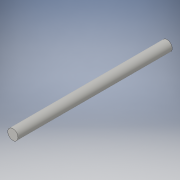
# Autodesk Inventor part: 4x40 Tap
Saved by Autodesk Inventor 2016 (Build 200138000, 138)
## iProperties
Created: 2015-09-21
Part Number: 4x40 Tap
Material: Generic
Document SubType Name: Modeling
Designer: steele
Density: 1 g/cm^3
Appearance: Default
Author: steele
Autodesk Inventor part; units mm, degrees
ref_plane "YZ Plane" through (0, 0, 0) normal (1, 0, 0) x (0, 1, 0)
ref_plane "XZ Plane" through (0, 0, 0) normal (0, 1, 0) x (-1, 0, 0)
ref_plane "XY Plane" through (0, 0, 0) normal (0, 0, 1) x (1, 0, 0)
sketch "Sketch1" plane through (0, 0, 0) normal (0, 0, 1) x (1, 0, 0)
  circle A0 centre (0, 0) radius 2.54
  dimension "d2" = 5.08
  constraints: 1 centre point, 1 coincident
  measures "d2" diameter of A0
extrude "Extrusion1" add sketch "Sketch1" along normal mid plane 76.2
equation "\"d2\" = tapDiam4x40"
equation "\"d0\" = tapLength4x40"
equation "\"tapDiam1d4x28\" = 5.08"
equation "\"tapDiam1d4x20\" = 5.08"
equation "\"tapDiam12x24\" = 5.08"
equation "\"tapDiam8x36\" = 5.08"
equation "\"tapDiam10x32\" = 5.08"
equation "\"tapLength4x40\" = 76.2"
equation "\"tapDiam8x32\" = 5.08"
equation "\"lowerCaseHeight\" = 127"
equation "\"tapDiam4x40\" = 5.08"
equation "\"fingerWidth\" = 19.05"
equation "\"lowerCaseDepth\" = 25.4"
equation "\"tapLength6x32\" = 76.2"
equation "\"lowerCaseWidth\" = 254"
equation "\"tapDiam12x28\" = 5.08"
equation "\"tapDiam6x32\" = 5.08"
equation "\"tapDiam6x40\" = 5.08"
equation "\"tapDiam10x24\" = 5.08"
equation "\"tapDiaam4x48\" = 5.08"
equation "\"tapLength4x48\" = 76.2"
body "Solid1"
